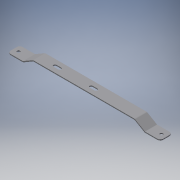
# Autodesk Inventor part: Part101
Saved by Autodesk Inventor 2016 (Build 200138000, 138)
## iProperties
Created: 2018-11-13
Part Number: Part101
Material: Generic
Document SubType Name: Sheet Metal
Designer: hovm
Density: 1 g/cm^3
Sheet Metal Rule: Default_mm
Appearance: Default
Author: hovm
Autodesk Inventor part; units mm, degrees
ref_plane "YZ Plane" through (0, 0, 0) normal (1, 0, 0) x (0, 1, 0)
ref_plane "XZ Plane" through (0, 0, 0) normal (0, 1, 0) x (-1, 0, 0)
ref_plane "XY Plane" through (0, 0, 0) normal (0, 0, 1) x (1, 0, 0)
sketch "Sketch1" plane through (0, 0, 0) normal (0, 0, 1) x (1, 0, 0)
  line L0 (-54.5, -12.5) -> (154.5, -12.5)
  line L1 (154.5, -12.5) -> (154.5, 12.5)
  line L2 (154.5, 12.5) -> (-54.5, 12.5)
  line L3 (-54.5, 12.5) -> (-54.5, -12.5)
  line L4 (-54.5, -12.5) -> (154.5, 12.5) construction
  line L5 (154.5, -12.5) -> (-54.5, 12.5) construction
  line L6 (149.5, 192.0914) -> (-150.5, 192.0914)
  line L7 (205, 191) -> (-105, 191)
  point P0 (50, 0)
  point P1 (50, 0)
  point P2 (50, 0)
  point P3 (50, 191)
  dimension "d0" = 25
  dimension "d1" = 209
  measures "d0" distance of L0.end L1.end
  measures "d1" distance of L1.end L2.end
extrude "Plate1" add sketch "Sketch1" along normal blind 2
sketch "Sketch2" plane through (153.5, -12.5, 0.2679) normal (0.5, 0, 0.8660254) x (0, 1, 0)
  line L0 (25, 0) -> (0, 0)
  line L1 (0, 0) -> (0, -25)
  line L2 (0, -25) -> (25, -25)
  line L3 (25, -25) -> (25, 0)
  constraints: 6 end point, 1 horizontal, 1 perpendicular, 1 vertical
edge flange "Flange1" height 25 angle 30 thickness 2 bend radius 2 thickness toward (0.5, 0, 0.8660254) relief tear relief width 2 relief depth 1 corner gap 2 corner form 0 edges at (154.5, 0, 0) (-54.5, 0, 0) wall of the first edge with corners at (153.5, 12.5, 0.2679) (153.5, -12.5, 0.2679) (175.1506, -12.5, -12.2321) (175.1506, 12.5, -12.2321)
bend "Bend1"
corner "Corner1"
sketch "Sketch3" plane through (175.1506, 12.5, -10.2321) normal (0, 0, -1) x (-1, 0, 0)
  line L0 (0, -25) -> (0, 0)
  line L1 (0, 0) -> (-29, 0)
  line L2 (-29, 0) -> (-29, -25)
  line L3 (-29, -25) -> (0, -25)
  constraints: 6 end point, 1 horizontal, 1 perpendicular, 1 vertical
edge flange "Flange2" height 29 angle 30 thickness 2 bend radius 2 thickness toward (0, 0, -1) relief tear relief width 2 relief depth 1 corner gap 2 corner form 0 edges at (176.1506, 0, -10.5) (-76.1506, 0, -10.5) wall of the first edge with corners at (175.1506, -12.5, -10.2321) (175.1506, 12.5, -10.2321) (204.1506, 12.5, -10.2321) (204.1506, -12.5, -10.2321)
bend "Bend2"
corner "Corner2"
sketch "Sketch4" plane through (0, 0, 2) normal (0, 0, 1) x (1, 0, 0)
  line L0 (-14.5, 0) -> (-4.5, 0) construction
  line L1 (-14.5, -3.2) -> (-4.5, -3.2)
  line L2 (-4.5, 3.2) -> (-14.5, 3.2)
  arc A0 (-14.5, 3.2) -> (-14.5, -3.2) centre (-14.5, 0) ccw
  arc A1 (-4.5, -3.2) -> (-4.5, 3.2) centre (-4.5, 0) ccw
  line L3 (60.5, 0) -> (70.5, 0) construction
  line L4 (60.5, -3.2) -> (70.5, -3.2)
  line L5 (70.5, 3.2) -> (60.5, 3.2)
  arc A2 (60.5, 3.2) -> (60.5, -3.2) centre (60.5, 0) ccw
  arc A3 (70.5, -3.2) -> (70.5, 3.2) centre (70.5, 0) ccw
  circle A4 centre (-9.5, 0) radius 3 projected
  circle A5 centre (65.5, 0) radius 2.3866 projected
  point P0 (0, 0)
  point P1 (-9.5, 0)
  point P2 (65.5, 0)
  dimension "d23" = 3.2
  dimension "d24" = 3.2
  dimension "d25" = 10
  dimension "d26" = 10
  constraints: 16 end point, 8 point on circle, 8 tangent, 4 centre point, 2 coincident, 2 midpoint, 2 parallel, 2 point on line, 1 horizontal, 1 horizontal alignment
  measures "d23" radius of A1
  measures "d24" radius of A3
  measures "d25" distance of L2.start L2.end
  measures "d26" distance of L5.start L5.end
extrude "Cut1" cut sketch "Sketch4" against normal blind 2 contours A0 L2 A1 L1 | A2 L5 A3 L4 | A4 | A5
sketch "Sketch5" plane through (-104.1506, -12.5, -10.2321) normal (0, 0, 1) x (1, 0, 0)
  line L0 (0, 25) -> (0, 0) projected
  line L1 (308.3013, 0) -> (308.3013, 25) projected
  circle A0 centre (300.8013, 12.5) radius 2.75 projected
  circle A1 centre (7.5, 12.5) radius 2.75 projected
  point P0 (104.1506, 12.5)
  point P1 (300.8013, 12.5)
  point P2 (0, 12.5)
  point P3 (308.3013, 12.5)
  constraints: 2 coincident, 2 horizontal alignment, 2 midpoint
hole "Hole1" at (-96.6506, 0, -10.2321) at (196.6506, 0, -10.2321) direction (0, 0, -1) diameter 7 depth 2 tip angle 118
fillet "Corner Round1" radius 6 4 edges at (-104.1506, 12.5, -11.2321) (-104.1506, -12.5, -11.2321) (204.1506, 12.5, -11.2321) (204.1506, -12.5, -11.2321)
equation "\"d27\" = Thickness"
equation "\"d36\" = Thickness"
equation "\"d3\" = BendReliefWidth"
equation "\"d4\" = BendReliefDepth"
equation "\"d5\" = MinimumRemnant"
equation "\"d6\" = BendRadius"
equation "\"d9\" = BendRadius"
equation "\"d10\" = CornerReliefSize"
equation "\"d11\" = GapSize"
equation "\"d12\" = JacobiRadiusSize"
equation "\"d13\" = BendReliefWidth"
equation "\"d14\" = BendReliefDepth"
equation "\"d15\" = MinimumRemnant"
equation "\"d16\" = BendRadius"
equation "\"d19\" = BendRadius"
equation "\"d20\" = CornerReliefSize"
equation "\"d21\" = GapSize"
equation "\"d22\" = JacobiRadiusSize"
equation "\"BendRadius\" = Thickness"
equation "\"BendReliefWidth\" = Thickness"
equation "\"BendReliefDepth\" = 0.5 * Thickness"
equation "\"CornerReliefSize\" = 4 * Thickness"
equation "\"MinimumRemnant\" = 2 * Thickness"
equation "\"TransitionRadius\" = BendRadius"
equation "\"JacobiRadiusSize\" = BendRadius"
equation "\"GapSize\" = Thickness"
equation "\"d2\" = BendRadius"
equation "\"Thickness\" = 2"
body "Solid1"
